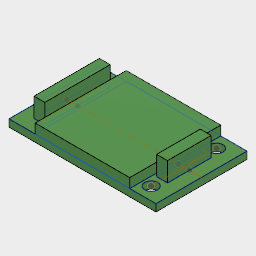
HX711 Breakout v2 (Autodesk Fusion 360 design; units mm, degrees)
Autodesk Fusion 360 part; units mm, degrees
sketch "Sketch1" plane through (0, 0, 0) normal (0, 1, 0) x (1, 0, 0)
  line L0 (-22.3654, 14.0021) -> (11.8346, 14.0021)
  line L1 (11.8346, 14.0021) -> (11.8346, -7.1979)
  line L2 (11.8346, -7.1979) -> (-22.3654, -7.1979)
  line L3 (-22.3654, -7.1979) -> (-22.3654, 14.0021)
  line L4 (-19.5354, 11.0221) -> (-16.9954, 11.0221)
  line L5 (-16.9954, 11.0221) -> (-16.9954, -4.2179)
  line L6 (-16.9954, -4.2179) -> (-19.5354, -4.2179)
  line L7 (-19.5354, -4.2179) -> (-19.5354, 11.0221)
  line L8 (6.4646, 8.4821) -> (9.0046, 8.4821)
  line L9 (9.0046, 8.4821) -> (9.0046, -1.6779)
  line L10 (9.0046, -1.6779) -> (6.4646, -1.6779)
  line L11 (6.4646, -1.6779) -> (6.4646, 8.4821)
  line L12 (11.8346, 3.4021) -> (-22.3654, 3.4021) construction
  line L13 (-16.2654, 14.0021) -> (5.7346, 14.0021)
  line L14 (5.7346, 14.0021) -> (5.7346, -7.1979)
  line L15 (5.7346, -7.1979) -> (-16.2654, -7.1979)
  line L16 (-16.2654, -7.1979) -> (-16.2654, 14.0021)
  line L17 (-18.2654, -4.2179) -> (-18.2654, 11.0221) construction
  line L18 (7.7346, -1.6779) -> (7.7346, 8.4821) construction
  circle A0 centre (7.7346, 11.0021) radius 1.5
  circle A1 centre (7.7346, -4.1979) radius 1.5
  line L19 (7.7346, -4.1979) -> (7.7346, 11.0021) construction
  point P0 (-16.9954, 3.4021)
  point P1 (-19.5354, 3.4021)
  point P2 (6.4646, 3.4021)
  point P3 (9.0046, 3.4021)
  dimension "d1" = 34.2
  dimension "d2" = 21.2
  dimension "d3" = 15.24
  dimension "d4" = 2.54
  dimension "d5" = 10.16
  dimension "d6" = 2.54
  dimension "d7" = 22
  dimension "d8" = 4.1
  dimension "d9" = 4.1
  dimension "d16" = 3
  dimension "d17" = 3
  dimension "d18" = 15.2
  measures "d1" distance of L0.start L0.end
  measures "d2" distance of L0.start L2.end
  measures "d3" distance of L4.start L6.end
  measures "d4" distance of L4.start L4.end
  measures "d5" distance of L8.start L10.end
  measures "d6" distance of L8.start L8.end
  measures "d7" distance of L13.start L13.end
  measures "d8" distance of L3 L17
  measures "d9" distance of L1 L18
  measures "d16" diameter of A0
  measures "d17" diameter of A1
  measures "d18" distance of A1.centre A0.centre
extrude "Extrude1" add sketch "Sketch1" against normal blind 1.7 contours L0 L2 L3 L16 | L0 L2 L13 L14 L15 L16 | L0 L1 L2 L14 | L4 L5 L6 L7 | L8 L9 L10 L11 | A0 | A1
extrude "Extrude2" add sketch "Sketch1" along normal blind 2.2 contours L0 L2 L13 L14 L15 L16
extrude "Extrude3" add sketch "Sketch1" along normal blind 4.5 contours L4 L5 L6 L7 | L8 L9 L10 L11
extrude "Extrude4" cut sketch "Sketch1" against normal blind 5 contours A0 | A1
